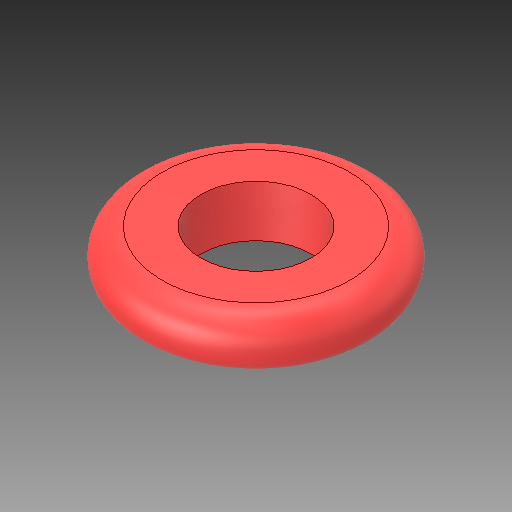
# Autodesk Inventor part: タミヤダンパー6
Saved by Autodesk Inventor 2020 (Build 240168000, 168)
## iProperties
Part Number: タミヤダンパー6
Material: ゴム
Document SubType Name: Modeling
Designer: 雪村
Density: 0.93 g/cm^3
Appearance: サテン - 淡い赤
Mass: 0.0301992 g
Surface Area: 0.813059 cm^2
Volume: 0.0324723 cm^3
Author: 雪村
Autodesk Inventor part; units mm, degrees
ref_plane "YZ Plane" through (0, 0, 0) normal (1, 0, 0) x (0, 1, 0)
ref_plane "XZ Plane" through (0, 0, 0) normal (0, 1, 0) x (-1, 0, 0)
ref_plane "XY Plane" through (0, 0, 0) normal (0, 0, 1) x (1, 0, 0)
sketch "スケッチ1" plane through (0, 0, 0) normal (0, 1, 0) x (-1, 0, 0)
  circle A0 centre (0, 0) radius 3.25
  circle A1 centre (0, 0) radius 1.5
  dimension "d0" = 6.5
  dimension "d1" = 3
  constraints: 2 centre point, 2 coincident
  measures "d0" diameter of A0
  measures "d1" diameter of A1
extrude "押し出し1" add sketch "スケッチ1" along normal blind 1.4
fillet "フィレット1" radius 0.7 2 edges at (3.25, 1.4, 0) (3.25, 0, 0)
